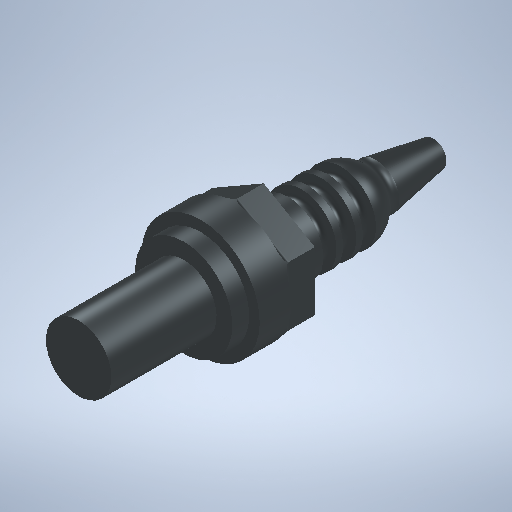
# Autodesk Inventor part: zündkerze
Saved by Autodesk Inventor 2025 (Build 290162010, 162A)
## iProperties
Created: 2024-07-15
Part Number: zündkerze
Material: Iron, Cast
Document SubType Name: Modeling
Designer: Fabri
Density: 7.15 g/cm^3
Appearance: Iron Gray
Author: Fabri
Autodesk Inventor part; units mm, degrees
ref_plane "XZ Plane" through (0, 0, 0) normal (0, 1, 0) x (-1, 0, 0)
sketch "Sketch1" plane through (0, 0, 0) normal (0, 1, 0) x (-1, 0, 0)
  line L0 (0, 4.5) -> (3.8971, 2.25)
  line L1 (3.8971, 2.25) -> (3.8971, -2.25)
  line L2 (3.8971, -2.25) -> (0, -4.5)
  line L3 (0, -4.5) -> (-3.8971, -2.25)
  line L4 (-3.8971, -2.25) -> (-3.8971, 2.25)
  line L5 (-3.8971, 2.25) -> (0, 4.5)
  point P0 (0, 0)
  point P1 (0, 0)
  dimension "d3" = 9
  constraints: 12 end point, 1 coincident, 13 other
  measures "d3" distance of L2.end L0.start
extrude "Extrusion1" add sketch "Sketch1" along normal blind 2.4
ref_plane "Work Plane1" through (0, 0, 0) normal (1, 0, 0) x (0, 1, 0)
sketch "Sketch2" plane through (0, 0, 0) normal (1, 0, 0) x (0, 1, 0)
  line L0 (0, 4.5) -> (-2.4, 4.5)
  line L1 (-2.4, 4.5) -> (-2.4, 3.7)
  line L2 (-2.4, 3.7) -> (-3.6814, 3.7)
  line L3 (-3.6814, 3.7) -> (-3.6814, 2.5)
  line L4 (-3.6814, 2.5) -> (-11.6814, 2.5)
  line L5 (-11.6814, 2.5) -> (-11.6814, 0)
  line L6 (-11.6814, 0) -> (0, 0)
  line L7 (2.4, 2.6755) -> (4.278, 2.6755)
  line L8 (4.278, 2.6755) -> (4.278, 1.75)
  line L9 (4.278, 1.75) -> (5.278, 1.75)
  line L10 (5.278, 1.75) -> (5.278, 2.6755)
  line L11 (5.278, 2.6755) -> (5.778, 2.6755)
  line L12 (5.778, 2.6755) -> (5.778, 1.75)
  line L13 (5.778, 1.75) -> (6.778, 1.75)
  line L14 (6.778, 1.75) -> (6.778, 2.6755)
  line L15 (6.778, 2.6755) -> (7.278, 2.6755)
  line L16 (7.278, 2.6755) -> (7.278, 1.75)
  line L17 (7.278, 1.75) -> (8.278, 1.75)
  line L18 (8.278, 1.75) -> (8.278, 2.6755)
  arc A0 (10.1076, 1.9521) -> (8.278, 2.6755) centre (8.278, 0) ccw
  arc A1 (10.1076, 1.9521) -> (10.9835, 1.75) centre (10.7195, 2.605) ccw
  line L19 (10.9835, 1.75) -> (15.3186, 1.0036)
  line L20 (15.3186, 1.0036) -> (15.3186, 0)
  line L21 (0, 0) -> (15.3186, 0)
  line L22 (2.4, 2.6755) -> (2.4, 0)
  line L23 (2.4, -2.25) -> (2.4, 2.25) projected
  line L24 (0, 4.5) -> (0, 0)
  line L25 (0, -2.25) -> (0, 2.25) projected
  point P0 (-1.2, 4.5)
  dimension "d7" = 8
  dimension "d8" = 5
  dimension "d9" = 7.4
  dimension "d10" = 9
  dimension "d12" = 27
  dimension "d14" = 1
  dimension "d15" = 1
  dimension "d16" = 1
  dimension "d17" = 3.5
  dimension "d18" = 5.351
  dimension "d19" = 0.5
  dimension "d20" = 0.5
  dimension "d21" = 2.4
  constraints: 48 end point, 12 perpendicular, 11 point on line, 5 horizontal alignment, 4 point on circle, 2 centre point, 2 horizontal, 2 midpoint, 1 collinear, 1 parallel, 1 tangent, 1 vertical alignment
  measures "d7" distance of L3.end L4.end
  measures "d8" diameter of L4 L6
  measures "d9" diameter of L2 L6
  measures "d10" diameter of point (-1.2, 4.5) L6
  measures "d12" distance between parallel lines of L20 L5
  measures "d14" distance between parallel lines of L10 L8
  measures "d15" distance between parallel lines of L18 L16
  measures "d16" distance between parallel lines of L14 L12
  measures "d17" diameter of L19.start L21
  measures "d18" diameter of L7.start L21
  measures "d19" distance of L14.end L15.end
  measures "d20" distance of L10.end L11.end
  measures "d21" distance of L0.start L0.end
revolve "Revolution1" add sketch "Sketch2" angle 360 about axis through (0, -11.6814, 0) along (0, 1, 0)
fillet "Fillet1" radius 0.45 6 edges at (0, 4.278, -1.75) (0, 5.278, -1.75) (0, 5.778, -1.75) (0, 6.778, -1.75) (0, 7.278, -1.75) (0, 8.278, -1.75)
fillet "Fillet2" radius 0.45 6 edges at (1.9486, 0, 3.375) (3.8971, 0, 0) (1.9486, 0, -3.375) (-1.9486, 0, -3.375) (-3.8971, 0, 0) (-1.9486, 0, 3.375)
ref_plane "Work Plane2" through (4.5, 0, 0) normal (1, 0, 0) x (0, 1, 0)
sketch "Sketch3" plane through (4.5, 0, 0) normal (1, 0, 0) x (0, 1, 0)
  line L0 (-11.6814, -2.5) -> (-11.6814, 2.5) projected
  circle A0 centre (-13.6814, 0) radius 0.25
  circle A1 centre (-13.6814, 0) radius 0.175
  point P0 (0, 0)
  point P1 (-11.6814, 0)
  dimension "d26" = 0.5
  dimension "d27" = 2
  dimension "d31" = 0.35
  constraints: 2 centre point, 1 coincident, 1 horizontal alignment, 1 midpoint
  measures "d26" diameter of A0
  measures "d27" distance from line of L0 A0.centre
  measures "d31" diameter of A1
sketch "Sketch4" plane through (0, 0, 0) normal (0, 0, 1) x (1, 0, 0)
  line L0 (4.5, -13.6814) -> (0.9966, -13.6814)
  arc A0 (0, -12.7635) -> (0.9966, -13.6814) centre (0.9966, -12.6814) ccw
  line L1 (0, -12.7635) -> (0, -11.6458)
  line L2 (2.5, -11.6814) -> (-2.5, -11.6814) projected
  point P0 (0, 0)
  point P1 (0, -11.6814)
  dimension "d28" = 1
  constraints: 4 end point, 2 point on circle, 1 centre point, 1 horizontal, 1 midpoint, 1 perpendicular, 1 tangent, 1 vertical alignment
  measures "d28" radius of A0
equation "\"d14\" = d15"
equation "\"d16\" = d15"
body "Solid1"
